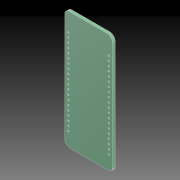
# Autodesk Inventor part: untitled.brdКонтур
Saved by Autodesk Inventor 2020 (Build 240168000, 168)
## iProperties
Created: 2021-08-05
Part Number: untitled.brdКонтур
Material: Типовые
Document SubType Name: Modeling
Designer: Петров Иван
Mass: 2.80573 g
Surface Area: 39.9985 cm^2
Volume: 2.80573 cm^3
Density: 1 g/cm^3
Appearance: Зеленый — полированный
Author: Петров Иван
Autodesk Inventor part; units mm, degrees
ref_plane "YZ Plane" through (0, 0, 0) normal (1, 0, 0) x (0, 1, 0)
ref_plane "XZ Plane" through (0, 0, 0) normal (0, 1, 0) x (-1, 0, 0)
ref_plane "XY Plane" through (0, 0, 0) normal (0, 0, 1) x (1, 0, 0)
sketch "Эскиз1" plane through (0, 0, 0) normal (0, 0, 1) x (1, 0, 0)
  line L0 (-0.992, 110.468) -> (-0.992, 49.381)
  line L1 (-0.992, 49.381) -> (-0.8881, 48.5921)
  line L2 (-0.8881, 48.5921) -> (-0.5836, 47.857)
  line L3 (-0.5836, 47.857) -> (-0.0993, 47.2257)
  line L4 (-0.0993, 47.2257) -> (0.532, 46.7414)
  line L5 (0.532, 46.7414) -> (1.2671, 46.4369)
  line L6 (1.2671, 46.4369) -> (2.056, 46.333)
  line L7 (2.056, 46.333) -> (23.9, 46.333)
  line L8 (23.9, 46.333) -> (24.4259, 46.4022)
  line L9 (24.4259, 46.4022) -> (24.916, 46.6052)
  line L10 (24.916, 46.6052) -> (25.3368, 46.9282)
  line L11 (25.3368, 46.9282) -> (25.6598, 47.349)
  line L12 (25.6598, 47.349) -> (25.8628, 47.8391)
  line L13 (25.8628, 47.8391) -> (25.932, 48.365)
  line L14 (25.932, 48.365) -> (25.932, 109.579)
  line L15 (25.932, 109.579) -> (25.8195, 110.4336)
  line L16 (25.8195, 110.4336) -> (25.4896, 111.23)
  line L17 (25.4896, 111.23) -> (24.9649, 111.9139)
  line L18 (24.9649, 111.9139) -> (24.281, 112.4386)
  line L19 (24.281, 112.4386) -> (23.4846, 112.7685)
  line L20 (23.4846, 112.7685) -> (22.63, 112.881)
  line L21 (22.63, 112.881) -> (1.421, 112.881)
  line L22 (1.421, 112.881) -> (0.7965, 112.7988)
  line L23 (0.7965, 112.7988) -> (0.2145, 112.5577)
  line L24 (0.2145, 112.5577) -> (-0.2852, 112.1742)
  line L25 (-0.2852, 112.1742) -> (-0.6687, 111.6745)
  line L26 (-0.6687, 111.6745) -> (-0.9098, 111.0925)
  line L27 (-0.9098, 111.0925) -> (-0.992, 110.468)
  circle A0 centre (-26.67, 99.06) radius 0.5
  circle A1 centre (-26.67, 96.52) radius 0.5
  circle A2 centre (-26.67, 93.98) radius 0.5
  circle A3 centre (-26.67, 91.44) radius 0.5
  circle A4 centre (-26.67, 104.14) radius 0.5
  circle A5 centre (-26.67, 88.9) radius 0.5
  circle A6 centre (-26.67, 86.36) radius 0.5
  circle A7 centre (-26.67, 106.68) radius 0.5
  circle A8 centre (-3.81, 63.5) radius 0.5
  circle A9 centre (-26.67, 83.82) radius 0.5
  circle A10 centre (-26.67, 81.28) radius 0.5
  circle A11 centre (-26.67, 78.74) radius 0.5
  circle A12 centre (-26.67, 76.2) radius 0.5
  circle A13 centre (-26.67, 73.66) radius 0.5
  circle A14 centre (-26.67, 71.12) radius 0.5
  circle A15 centre (-26.67, 68.58) radius 0.5
  circle A16 centre (-26.67, 66.04) radius 0.5
  circle A17 centre (-26.67, 63.5) radius 0.5
  circle A18 centre (-26.67, 60.96) radius 0.5
  circle A19 centre (-3.81, 88.9) radius 0.5
  circle A20 centre (-3.81, 86.36) radius 0.5
  circle A21 centre (-3.81, 83.82) radius 0.5
  circle A22 centre (-3.81, 81.28) radius 0.5
  circle A23 centre (-3.81, 78.74) radius 0.5
  circle A24 centre (-3.81, 76.2) radius 0.5
  circle A25 centre (-3.81, 73.66) radius 0.5
  circle A26 centre (-3.81, 71.12) radius 0.5
  circle A27 centre (-3.81, 68.58) radius 0.5
  circle A28 centre (-3.81, 66.04) radius 0.5
  circle A29 centre (-3.81, 60.96) radius 0.5
  circle A30 centre (-3.81, 96.52) radius 0.5
  circle A31 centre (-26.67, 101.6) radius 0.5
  circle A32 centre (-3.81, 104.14) radius 0.5
  circle A33 centre (-3.81, 101.6) radius 0.5
  circle A34 centre (-3.81, 91.44) radius 0.5
  circle A35 centre (-26.67, 109.22) radius 0.5
  circle A36 centre (-3.81, 99.06) radius 0.5
  circle A37 centre (-3.81, 109.22) radius 0.5
  circle A38 centre (-3.81, 106.68) radius 0.5
  circle A39 centre (-3.81, 93.98) radius 0.5
  circle A40 centre (1.02, 92.33) radius 0.5
  circle A41 centre (1.02, 89.79) radius 0.5
  circle A42 centre (1.02, 87.25) radius 0.5
  circle A43 centre (1.02, 84.71) radius 0.5
  circle A44 centre (1.02, 97.41) radius 0.5
  circle A45 centre (1.02, 82.17) radius 0.5
  circle A46 centre (1.02, 79.63) radius 0.5
  circle A47 centre (1.02, 99.95) radius 0.5
  circle A48 centre (23.88, 56.77) radius 0.5
  circle A49 centre (1.02, 77.09) radius 0.5
  circle A50 centre (1.02, 74.55) radius 0.5
  circle A51 centre (1.02, 72.01) radius 0.5
  circle A52 centre (1.02, 69.47) radius 0.5
  circle A53 centre (1.02, 66.93) radius 0.5
  circle A54 centre (1.02, 64.39) radius 0.5
  circle A55 centre (1.02, 61.85) radius 0.5
  circle A56 centre (1.02, 59.31) radius 0.5
  circle A57 centre (1.02, 56.77) radius 0.5
  circle A58 centre (1.02, 54.23) radius 0.5
  circle A59 centre (23.88, 82.17) radius 0.5
  circle A60 centre (23.88, 79.63) radius 0.5
  circle A61 centre (23.88, 77.09) radius 0.5
  circle A62 centre (23.88, 74.55) radius 0.5
  circle A63 centre (23.88, 72.01) radius 0.5
  circle A64 centre (23.88, 69.47) radius 0.5
  circle A65 centre (23.88, 66.93) radius 0.5
  circle A66 centre (23.88, 64.39) radius 0.5
  circle A67 centre (23.88, 61.85) radius 0.5
  circle A68 centre (23.88, 59.31) radius 0.5
  circle A69 centre (23.88, 54.23) radius 0.5
  circle A70 centre (23.88, 89.79) radius 0.5
  circle A71 centre (1.02, 94.87) radius 0.5
  circle A72 centre (23.88, 97.41) radius 0.5
  circle A73 centre (23.88, 94.87) radius 0.5
  circle A74 centre (23.88, 84.71) radius 0.5
  circle A75 centre (1.02, 102.49) radius 0.5
  circle A76 centre (23.88, 92.33) radius 0.5
  circle A77 centre (23.88, 102.49) radius 0.5
  circle A78 centre (23.88, 99.95) radius 0.5
  circle A79 centre (23.88, 87.25) radius 0.5
  constraints: 80 centre point, 56 end point
extrude "untitled.brdКонтур" add sketch "Эскиз1" along normal blind 1.6
sketch "Эскиз2" plane through (-0.992, 49.381, 0) normal (-1, 0, 0) x (0, 0, 1)
  line L0 (-26.1671, -21.9018) -> (16.6735, -21.9018)
  line L1 (16.6735, -21.9018) -> (16.6735, 72.0181)
  line L2 (16.6735, 72.0181) -> (-26.1671, 72.0181)
  line L3 (-26.1671, 72.0181) -> (-26.1671, -21.9018)
  point P0 (0, -49.381)
  constraints: 8 end point, 2 parallel, 1 horizontal, 1 perpendicular
extrude "Выдавливание2" cut sketch "Эскиз2" along normal blind 30.75
